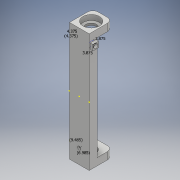
# Autodesk Inventor part: mtv_frontAxelHolder(4_30)
Saved by Autodesk Inventor 2018 (Build 220112000, 112)
## iProperties
Created: 2019-04-30
Part Number: mtv_frontAxelHolder(4_30)
Material: Generic
Document SubType Name: Modeling
Designer: Aditya Kendre
Density: 1 g/cm^3
Appearance: Default
Author: Aditya Kendre
## iProperties of the stored document mtv_frontAxelHolder(4_30)_3DPrint.ipt
Created: 2019-04-30
Part Number: mtv_frontAxelHolder(4_30)_3DPrint
Material: Generic
Document SubType Name: Modeling
Designer: Aditya Kendre
Density: 1 g/cm^3
Appearance: Default
Author: Aditya Kendre
Autodesk Inventor part; units mm, degrees
ref_plane "YZ Plane" through (0, 0, 0) normal (1, 0, 0) x (0, 1, 0)
ref_plane "XZ Plane" through (0, 0, 0) normal (0, 1, 0) x (-1, 0, 0)
ref_plane "XY Plane" through (0, 0, 0) normal (0, 0, 1) x (1, 0, 0)
sketch "Sketch1" plane through (0, 0, 0) normal (0, 1, 0) x (-1, 0, 0)
  line L0 (-6.985, 50) -> (6.985, 50)
  line L1 (6.985, 50) -> (6.985, -50)
  line L2 (6.985, -50) -> (-6.985, -50)
  line L3 (-6.985, -50) -> (-6.985, 50)
  line L4 (-6.985, 50) -> (6.985, -50) construction
  line L5 (6.985, 50) -> (-6.985, -50) construction
  point P0 (0, 0)
  dimension "d0" = 13.97
  dimension "d1" = 100
  constraints: 12 end point, 2 midpoint, 2 parallel, 1 horizontal, 1 perpendicular
  measures "d0" distance of L1.end L2.end
  measures "d1" distance of L0.end L1.end
extrude "Extrusion1" add sketch "Sketch1" along normal blind 2
sketch "Sketch2" plane through (0, 0, 0) normal (0, -1, 0) x (1, 0, 0)
  point P0 (0, 0)
sketch "Sketch3" plane through (0, 2, 0) normal (0, 1, 0) x (1, 0, 0)
  point P0 (0, 0)
sketch "Sketch4" plane through (0, 0, 0) normal (0, -1, 0) x (1, 0, 0)
  line L0 (6.985, -50) -> (-6.985, -50) projected
  line L1 (-6.985, -50) -> (-9.485, -50)
  line L2 (-9.485, -50) -> (-9.485, 50)
  line L3 (-9.485, 50) -> (-6.985, 50)
  line L4 (-6.985, 50) -> (-6.985, -50)
  line L5 (-6.985, 50) -> (6.985, 50) projected
  line L6 (6.985, 50) -> (9.485, 50)
  line L7 (9.485, 50) -> (9.485, -50)
  line L8 (9.485, -50) -> (6.985, -50)
  line L9 (6.985, -50) -> (6.985, 50)
  point P0 (0, 0)
  dimension "d4" = 2.5
  dimension "d5" = 2.5
  constraints: 16 end point, 4 parallel, 2 horizontal, 2 perpendicular, 1 point on line
  measures "d4" distance of L2.end L3.end
  measures "d5" distance of L7.end L8.end
extrude "Extrusion2" add sketch "Sketch4" against normal blind 10.89 contours L9 L6 L7 L8 | L1 L2 L3 L4
sketch "Sketch5" plane through (0, 10.89, 0) normal (0, 1, 0) x (1, 0, 0)
  line L0 (9.485, 50) -> (9.485, -50) projected
  line L1 (6.985, 50) -> (-6.985, 50) projected
  line L2 (9.485, -50) -> (6.985, -50)
  line L3 (6.985, -50) -> (6.985, 50)
  line L4 (6.985, 50) -> (9.485, 50)
  line L5 (9.485, 50) -> (9.485, -50)
  point P0 (0, 0)
  constraints: 8 end point, 2 parallel, 1 horizontal, 1 perpendicular
extrude "Extrusion3" cut sketch "Sketch5" against normal blind 3.14
sketch "Sketch6" plane through (0, 10.89, 0) normal (0, 1, 0) x (1, 0, 0)
  line L0 (-6.985, 50) -> (-6.985, -50) projected
  line L1 (-9.485, -50) -> (-9.485, 50) projected
  line L2 (-6.985, -50) -> (-9.485, -50)
  line L3 (-9.485, -50) -> (-9.485, 50)
  line L4 (-9.485, 50) -> (-6.985, 50)
  line L5 (-6.985, 50) -> (-6.985, -50)
  point P0 (0, 0)
  constraints: 8 end point, 2 parallel, 1 horizontal, 1 perpendicular
extrude "Extrusion4" cut sketch "Sketch6" against normal blind 2.14
sketch "Sketch7" plane through (0, 8.75, 0) normal (0, 1, 0) x (1, 0, 0)
  line L0 (-6.985, 50) -> (-6.985, -50) projected
  line L1 (-9.485, -50) -> (-9.485, 50) projected
  line L2 (-6.985, 0) -> (-9.485, 0)
  line L3 (-9.485, 0) -> (-9.485, 3.5)
  line L4 (-9.485, 3.5) -> (-6.985, 3.5)
  line L5 (-6.985, 3.5) -> (-6.985, 0)
  point P0 (0, 0)
  dimension "d12" = 3.5
  constraints: 8 end point, 2 parallel, 1 horizontal, 1 midpoint, 1 perpendicular, 1 point on line
  measures "d12" distance of L2.end L3.end
extrude "Extrusion5" add sketch "Sketch7" along normal blind 2.14
fillet "Fillet1" radius 7 2 edges at (-8.235, 8.75, -3.5) (-8.235, 10.89, -3.5)
sketch "Sketch8" plane through (-9.485, 0, 50) normal (0, 0, 1) x (1, 0, 0)
  line L0 (0, 0) -> (0, 8.75) construction
  line L1 (0, 0) -> (18.97, 0) construction
  line L2 (18.97, 0) -> (18.97, 11.43) construction
  line L3 (18.97, 11.43) -> (0, 11.43) construction
  line L4 (0, 11.43) -> (0, 0) construction
  line L5 (0, 0) -> (18.97, 0)
  line L6 (18.97, 0) -> (18.97, 22.5)
  line L7 (18.97, 22.5) -> (0, 22.5)
  line L8 (0, 22.5) -> (0, 0)
  circle A0 centre (9.485, 11.43) radius 7.9875
  point P0 (9.485, 0)
  dimension "d16" = 11.43
  dimension "d17" = 22.5
  dimension "d18" = 15.975
  constraints: 16 end point, 4 parallel, 2 horizontal, 2 perpendicular, 1 centre point, 1 coincident, 1 midpoint, 1 point on line
  measures "d16" distance of L2.end L1.end
  measures "d17" distance of L6.end L5.end
  measures "d18" diameter of A0
extrude "Extrusion6" add sketch "Sketch8" along normal blind 7
sketch "Sketch9" plane through (9.485, 0, -50) normal (0, 0, -1) x (-1, 0, 0)
  line L0 (0, 22.5) -> (18.97, 22.5) projected
  line L1 (0, 0) -> (18.97, 0)
  line L2 (18.97, 0) -> (18.97, 22.5)
  line L3 (18.97, 22.5) -> (0, 22.5)
  line L4 (0, 22.5) -> (0, 0)
  circle A0 centre (9.485, 11.43) radius 7.9875 projected
  circle A1 centre (9.485, 11.43) radius 7.9875
  point P0 (9.485, 0)
  constraints: 8 end point, 2 parallel, 1 centre point, 1 coincident, 1 horizontal, 1 perpendicular
extrude "Extrusion7" add sketch "Sketch9" along normal blind 7
fillet "Fillet2" radius 5 4 edges at (-9.485, 22.5, -53.5) (9.485, 22.5, 53.5) (-9.485, 22.5, 53.5) (9.485, 22.5, -53.5)
sketch "Sketch10" plane through (-9.485, 0, 50) normal (0, 0, -1) x (-1, 0, 0)
  circle A0 centre (-9.485, 11.43) radius 7.9875 projected
  circle A1 centre (-9.485, 11.43) radius 7.9875
  circle A2 centre (-9.485, 11.43) radius 3.175 construction
  circle A3 centre (-9.485, 11.43) radius 5
  point P0 (-9.485, 0)
  dimension "d24" = 6.35
  dimension "d25" = 10
  constraints: 3 centre point, 3 coincident
  measures "d24" diameter of A2
  measures "d25" diameter of A3
extrude "Extrusion8" add sketch "Sketch10" against normal blind 2
sketch "Sketch11" plane through (9.485, 0, -50) normal (0, 0, 1) x (1, 0, 0)
  circle A0 centre (-9.485, 11.43) radius 5 projected
  circle A1 centre (-9.485, 11.43) radius 7.9875
  circle A2 centre (-9.485, 11.43) radius 5
  point P0 (-9.485, 0)
  dimension "d28" = 10
  constraints: 2 centre point, 2 coincident
  measures "d28" diameter of A2
extrude "Extrusion9" add sketch "Sketch11" against normal blind 2
sketch "Sketch12" plane through (0, 8.75, 0) normal (0, 1, 0) x (1, 0, 0)
  point P0 (0, 0)
sketch "Sketch13" plane through (0, 2, 0) normal (0, 1, 0) x (1, 0, 0)
  line L0 (6.985, 50) -> (-6.985, 50) construction
  line L1 (-6.985, 50) -> (-6.985, 8.5379) construction
  line L2 (6.985, 50) -> (-6.985, 50) construction
  line L3 (-6.985, 50) -> (-6.985, 36.03) construction
  line L4 (-6.985, 36.03) -> (6.985, 36.03) construction
  line L5 (6.985, 36.03) -> (6.985, 50) construction
  circle A0 centre (0, 43.015) radius 1.5875
  point P0 (0, 0)
  dimension "d31" = 13.97
  dimension "d32" = 3.175
  constraints: 8 end point, 2 parallel, 1 centre point, 1 coincident, 1 horizontal, 1 perpendicular, 1 point on line
  measures "d31" distance of L3.end L2.end
  measures "d32" diameter of A0
extrude "Extrusion10" cut sketch "Sketch13" against normal blind 2
fillet "Fillet3" radius 2 1 edges at (-1.5875, 2, -43.015)
sketch "Sketch14" plane through (0, 2, 0) normal (0, 1, 0) x (1, 0, 0)
  circle A0 centre (0, 43.015) radius 1.5875 construction
  line L0 (0, 43.015) -> (-9.485, 43.015) construction
  line L1 (-9.485, 8.5379) -> (-9.485, 50) construction
  line L2 (0, 43.015) -> (0, 50) construction
  line L3 (6.985, 50) -> (-6.985, 50) construction
  point P0 (0, 0)
  dimension "d36" = 6.985
  dimension "d37" = 9.485
  constraints: 4 end point, 1 horizontal, 1 midpoint, 1 point on line
  measures "d36" distance of L0.start L2.end
  measures "d37" distance of L0.start L0.end
sketch "Sketch15" plane through (-9.485, 8.75, 0) normal (-1, 0, 0) x (0, 0, 1)
  point P0 (0, -8.75)
sketch "Sketch16" plane through (9.485, 0, 57) normal (1, 0, 0) x (0, 0, -1)
  line L0 (107, 7.75) -> (7, 7.75) construction
  line L1 (114, 0) -> (0, 0) construction
  line L2 (7, 7.75) -> (14.75, 7.75) construction
  line L3 (14.75, 7.75) -> (14.75, 0) construction
  line L4 (14.75, 0) -> (7, 0) construction
  line L5 (7, 0) -> (7, 7.75) construction
  line L6 (13.625, 1.125) -> (8.125, 1.125)
  line L7 (8.125, 1.125) -> (8.125, 6.625)
  line L8 (8.125, 6.625) -> (13.625, 6.625)
  line L9 (13.625, 6.625) -> (13.625, 1.125)
  line L10 (13.625, 1.125) -> (8.125, 6.625) construction
  line L11 (8.125, 1.125) -> (13.625, 6.625) construction
  circle A0 centre (10.875, 3.875) radius 2
  point P0 (57, 0)
  dimension "d38" = 7.75
  dimension "d39" = 5.5
  dimension "d40" = 5.5
  dimension "d41" = 4
  constraints: 20 end point, 4 parallel, 2 horizontal, 2 midpoint, 2 perpendicular, 1 centre point, 1 coincident, 1 point on line
  measures "d38" distance of L3.end L4.end
  measures "d39" distance of L7.end L8.end
  measures "d40" distance of L6.end L7.end
  measures "d41" diameter of A0
extrude "Extrusion11" add sketch "Sketch16" along normal blind 2.5
sketch "Sketch17" plane through (9.485, 3.875, 46.125) normal (1, 0, 0) x (0, 0, -1)
  circle A0 centre (0, 0) radius 2 construction
  line L0 (0, 0) -> (-3.875, 0) construction
  line L1 (-3.875, 0) -> (-3.875, -3.875) construction
  line L2 (-3.875, -3.875) -> (0, -3.875) construction
  line L3 (0, -3.875) -> (0, 0) construction
  point P0 (46.125, -3.875)
  dimension "d44" = 3.875
  dimension "d45" = 3.875
  constraints: 8 end point, 2 parallel, 1 horizontal, 1 perpendicular
  measures "d44" distance of L0.start L0.end
  measures "d45" distance of L2.end L0.start
sketch "Sketch18" plane through (0, 0, 0) normal (0, -1, 0) x (1, 0, 0)
  point P0 (0, 0)
sketch "Sketch19" plane through (-9.485, 8.75, 0) normal (-1, 0, 0) x (0, 0, 1)
  point P0 (0, -8.75)
sketch "Sketch20" plane through (-9.485, 8.75, 0) normal (-1, 0, 0) x (0, 0, 1)
  line L0 (50, -2.32) -> (50, 7.68) construction
  line L1 (-57, -8.75) -> (57, -8.75) construction
  line L2 (50, 0) -> (41.25, 0) construction
  line L3 (41.25, 0) -> (41.25, -8.75) construction
  line L4 (41.25, -8.75) -> (50, -8.75) construction
  line L5 (50, -8.75) -> (50, 0) construction
  circle A0 centre (45.625, -4.375) radius 1.5 construction
  circle A1 centre (45.625, -4.375) radius 1.5
  point P0 (0, -8.75)
  dimension "d46" = 8.75
  dimension "d47" = 3
  constraints: 8 end point, 2 centre point, 2 parallel, 2 point on line, 1 coincident, 1 horizontal, 1 perpendicular
  measures "d46" distance of L4.end L3.end
  measures "d47" diameter of A0
extrude "Extrusion12" add sketch "Sketch20" along normal blind 3
sketch "Sketch21" plane through (-9.485, 8.75, 0) normal (-1, 0, 0) x (0, 0, 1)
  circle A0 centre (45.625, -4.375) radius 1.5 construction
  line L0 (45.625, -4.375) -> (50, -4.375) construction
  line L1 (57, -8.75) -> (-57, -8.75) construction
  line L2 (45.625, -4.375) -> (50, -4.375) construction
  line L3 (50, -4.375) -> (50, -8.75) construction
  line L4 (50, -8.75) -> (45.625, -8.75) construction
  line L5 (45.625, -8.75) -> (45.625, -4.375) construction
  point P0 (0, -8.75)
  point P1 (50, 0)
  dimension "d50" = 4.375
  dimension "d51" = 4.375
  constraints: 10 end point, 2 horizontal, 2 parallel, 1 perpendicular, 1 point on line
  measures "d50" distance of L0.start L0.end
  measures "d51" distance of L4.end L0.start
body "Solid1"
